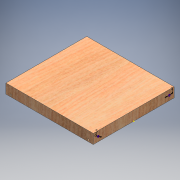
# Autodesk Inventor part: 240626_tablep1
Saved by Autodesk Inventor 2016 (Build 200138000, 138)
## iProperties
Created: 2024-06-26
Part Number: 240626_tablep1
Material: 일반
Document SubType Name: Modeling
Designer: pc
Density: 1 g/cm^3
Appearance: 자작나무 - 내츄럴 연마
Author: pc
Autodesk Inventor part; units mm, degrees
ref_plane "YZ Plane" through (0, 0, 0) normal (1, 0, 0) x (0, 1, 0)
ref_plane "XZ Plane" through (0, 0, 0) normal (0, 1, 0) x (-1, 0, 0)
ref_plane "XY Plane" through (0, 0, 0) normal (0, 0, 1) x (1, 0, 0)
sketch "스케치1" plane through (0, 0, 0) normal (0, 0, 1) x (1, 0, 0)
  line L0 (135, -125) -> (-135, -125)
  line L1 (-135, -125) -> (-135, 125)
  line L2 (-135, 125) -> (135, 125)
  line L3 (135, 125) -> (135, -125)
  line L4 (135, -125) -> (-135, 125) construction
  line L5 (-135, -125) -> (135, 125) construction
  point P0 (0, 0)
  dimension "d0" = 270
  dimension "d1" = 250
  constraints: 12 end point, 2 midpoint, 2 parallel, 1 horizontal, 1 perpendicular
  measures "d0" distance of L1.end L2.end
  measures "d1" distance of L0.end L1.end
extrude "돌출1" add sketch "스케치1" along normal blind 30
sketch "스케치2" plane through (-135, -125, 0) normal (0, -1, 0) x (1, 0, 0)
  circle A0 centre (15, 5.5) radius 2.5
  line L0 (270, 0) -> (0, 0) projected
  circle A1 centre (255, 5.5) radius 2.5
  line L1 (0, 0) -> (0, 30) projected
  line L2 (270, 0) -> (270, 30) projected
  point P0 (135, 0)
  dimension "d4" = 5
  dimension "d6" = 3
  dimension "d7" = 5
  dimension "d8" = 15
  dimension "d9" = 15
  constraints: 2 centre point
  measures "d4" diameter of A0
  measures "d6" distance edge to line of A0 L0
  measures "d7" diameter of A1
  measures "d8" distance from line of L1 A0.centre
  measures "d9" distance from line of L2 A1.centre
extrude "돌출2" cut sketch "스케치2" against normal blind 30
sketch "스케치3" plane through (-135, -125, 0) normal (-1, 0, 0) x (0, 0, 1)
  circle A0 centre (15, 235) radius 2.5
  circle A1 centre (15, 15) radius 2.5
  line L0 (0, 0) -> (30, 0) projected
  line L1 (0, 0) -> (0, 250) projected
  line L2 (0, 250) -> (30, 250) projected
  point P0 (0, 125)
  dimension "d12" = 5
  dimension "d13" = 5
  dimension "d14" = 15
  dimension "d15" = 15
  dimension "d16" = 15
  dimension "d17" = 15
  constraints: 2 centre point
  measures "d12" diameter of A0
  measures "d13" diameter of A1
  measures "d14" distance from line of L0 A1.centre
  measures "d15" distance from line of L1 A1.centre
  measures "d16" distance from line of L2 A0.centre
  measures "d17" distance from line of L1 A0.centre
extrude "돌출3" cut sketch "스케치3" against normal blind 30
sketch "스케치4" plane through (-135, 125, 0) normal (0, 1, 0) x (1, 0, 0)
  circle A0 centre (260, -5) radius 2.5
  circle A1 centre (10, -5) radius 2.5
  line L0 (0, 0) -> (270, 0) projected
  line L1 (270, 0) -> (270, -30) projected
  line L2 (0, 0) -> (0, -30) projected
  point P0 (135, 0)
  dimension "d20" = 5
  dimension "d21" = 5
  dimension "d22" = 5
  dimension "d23" = 10
  dimension "d24" = 10
  dimension "d25" = 5
  constraints: 2 centre point
  measures "d20" diameter of A0
  measures "d21" diameter of A1
  measures "d22" distance from line of L0 A0.centre
  measures "d23" distance from line of L1 A0.centre
  measures "d24" distance from line of L2 A1.centre
  measures "d25" distance from line of L0 A1.centre
extrude "돌출4" cut sketch "스케치4" against normal blind 30
sketch "스케치5" plane through (135, -125, 0) normal (1, 0, 0) x (0, 0, -1)
  circle A0 centre (-15, 15) radius 2.5 projected
  circle A1 centre (-15, 15) radius 2.5
  circle A2 centre (-15, 235) radius 2.5 projected
  circle A3 centre (-15, 235) radius 2.5
  point P0 (0, 125)
  dimension "d28" = 5
  dimension "d29" = 5
  constraints: 2 centre point, 2 coincident
  measures "d28" diameter of A1
  measures "d29" diameter of A3
extrude "돌출5" cut sketch "스케치5" against normal blind 30 contours A2
extrude "돌출6" cut sketch "스케치5" against normal blind 30 contours A0
